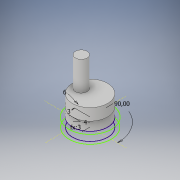
# Autodesk Inventor part: ExcentricShaft
Saved by Autodesk Inventor 2018.3 (Build 223284000, 284)
## iProperties
Created: 2018-07-20
Part Number: ExcentricShaft
Material: Generisch
Document SubType Name: Modeling
Designer: JochenAlt
Density: 1 g/cm^3
Appearance: Vorgabe
Author: JochenAlt
Autodesk Inventor part; units mm, degrees
ref_plane "YZ Plane" through (0, 0, 0) normal (1, 0, 0) x (0, 1, 0)
ref_plane "XZ Plane" through (0, 0, 0) normal (0, 1, 0) x (-1, 0, 0)
ref_plane "XY Plane" through (0, 0, 0) normal (0, 0, 1) x (1, 0, 0)
sketch "Skizze1" plane through (0, 0, 0) normal (0, 0, 1) x (1, 0, 0)
  line L0 (0, 15.4794) -> (0, -12.4794) construction
  line L1 (-12.4794, 0) -> (15.4794, 0) construction
  circle A0 centre (0, 0) radius 2
  arc A1 (-2.4686, -2.4686) -> (5.4686, 5.4686) centre (3, 0) ccw
  line L2 (0, -3) -> (0, 0) construction
  line L3 (0, 0) -> (3, 0) construction
  arc A2 (5.4686, 5.4686) -> (-2.4686, -2.4686) centre (0, 3) ccw
  arc A3 (-2.4686, -2.4686) -> (5.4686, 5.4686) centre (0, 3) ccw
  arc A4 (5.4686, 5.4686) -> (-2.4686, -2.4686) centre (3, 0) ccw
  circle A5 centre (3, 0) radius 7.1888
  circle A6 centre (0, 3) radius 7.2715
  line L4 (0, 0) -> (0, 8.4757) construction
  dimension "d0" = 4
  dimension "d1" = 3
  dimension "d13" = 6
  dimension "d16" = 90
  dimension "d17" = 3
  constraints: 9 point on circle, 7 centre point, 6 end point, 3 coincident, 3 equal radius, 2 collinear, 2 point on line, 1 concentric, 1 perpendicular
  measures "d0" diameter of A0
  measures "d1" distance of point (0, 0) A2.centre
  measures "d13" radius of A2
  measures "d16" angle of L4 L1
  measures "d17" distance of point (0, 0) L3.end
extrude "Extrusion2" add sketch "Skizze1" along normal blind 4 contours A0 | A4 A3 | A2 A5 A4 | A2 A5
extrude "Extrusion3" add sketch "Skizze1" along normal blind 2 from surface at 4 contours A0 | A4 A3
extrude "Extrusion4" add sketch "Skizze1" along normal blind 4 from surface at 6 contours A0 | A3 A1 A6 | A4 A3 | A6 A1
extrude "Extrusion5" add sketch "Skizze1" along normal blind 10 from surface at 10 contours A0
extrude "Extrusion6" add sketch "Skizze1" against normal blind 1 contours A0
equation "\"d17\" = d1"
